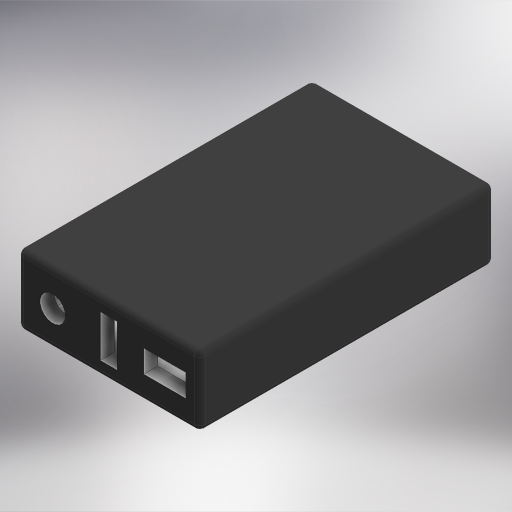
# Autodesk Inventor part: Lithium Battery
Saved by Autodesk Inventor 2024 (Build 280153000, 153)
## iProperties
Created: 2023-11-02
Part Number: Lithium Battery
Material: Genérico
Document SubType Name: Modeling
Designer: juesr
Density: 1 g/cm^3
Appearance: Valor por defecto
Author: juesr
Autodesk Inventor part; units mm, degrees
ref_plane "YZ Plane" through (0, 0, 0) normal (1, 0, 0) x (0, 1, 0)
ref_plane "XZ Plane" through (0, 0, 0) normal (0, 1, 0) x (-1, 0, 0)
ref_plane "XY Plane" through (0, 0, 0) normal (0, 0, 1) x (1, 0, 0)
sketch "Boceto1" plane through (0, 0, 0) normal (0, 1, 0) x (-1, 0, 0)
  line L0 (1.7308, 43.9183) -> (-63.2692, 43.9183)
  line L1 (-63.2692, 43.9183) -> (-63.2692, -61.0817)
  line L2 (-63.2692, -61.0817) -> (1.7308, -61.0817)
  line L3 (1.7308, -61.0817) -> (1.7308, 43.9183)
  point P0 (0, 0)
  dimension "d0" = 105
  dimension "d1" = 65
  constraints: 8 end point, 2 parallel, 1 horizontal, 1 perpendicular
  measures "d0" distance between parallel lines of L2 L0
  measures "d1" distance between parallel lines of L1 L3
extrude "Extrusión1" add sketch "Boceto1" along normal blind 25
shell "Vaciado1" thickness 5 removed faces 1 at (19.9359, 25, -26.0817)
sketch "Boceto2" plane through (0, 25, 0) normal (0, 1, 0) x (1, 0, 0)
  line L0 (3.2692, 56.0817) -> (3.2692, -38.9183) projected
  line L1 (58.2692, 56.0817) -> (3.2692, 56.0817)
  line L2 (3.2692, 56.0817) -> (3.2692, -38.9183)
  line L3 (3.2692, -38.9183) -> (58.2692, -38.9183)
  line L4 (58.2692, -38.9183) -> (58.2692, 56.0817)
  point P0 (0, 0)
  constraints: 8 end point, 2 parallel, 1 horizontal, 1 perpendicular
extrude "Extrusión2" add sketch "Boceto2" against normal blind 5
sketch "Boceto3" plane through (-1.7308, 0, 43.9183) normal (0, 0, 1) x (1, 0, 0)
  circle A0 centre (12.5, 12.5) radius 4.5
  line L0 (0, 0) -> (65, 0) projected
  line L1 (0, 0) -> (0, 25) projected
  point P0 (1.7308, 0)
  dimension "d12" = 9
  dimension "d13" = 12.5
  dimension "d14" = 12.5
  constraints: 1 centre point
  measures "d12" diameter of A0
  measures "d13" distance from line of L0 A0.centre
  measures "d14" distance from line of L1 A0.centre
extrude "Extrusión3" cut sketch "Boceto3" against normal blind 5
sketch "Boceto4" plane through (-1.7308, 0, 43.9183) normal (0, 0, 1) x (1, 0, 0)
  line L0 (60, 20) -> (5, 20) projected
  line L1 (60, 5) -> (5, 5) projected
  line L2 (29.5, 20) -> (35.5, 20)
  line L3 (35.5, 20) -> (35.5, 5)
  line L4 (35.5, 5) -> (29.5, 5)
  line L5 (29.5, 5) -> (29.5, 20)
  line L6 (0, 0) -> (0, 25) projected
  line L7 (65, 0) -> (65, 25) projected
  point P0 (1.7308, 0)
  point P1 (29.5, 12.5)
  point P2 (0, 12.5)
  dimension "d17" = 6
  dimension "d18" = 29.5
  dimension "d19" = 29.5
  constraints: 8 end point, 2 midpoint, 2 parallel, 2 point on line, 1 horizontal, 1 perpendicular
  measures "d17" distance from line of L3 point (29.5, 12.5)
  measures "d18" distance from line of point (0, 12.5) L5
  measures "d19" distance between parallel lines of L7 L3
extrude "Extrusión4" cut sketch "Boceto4" against normal blind 5
sketch "Boceto5" plane through (-1.7308, 0, 43.9183) normal (0, 0, 1) x (1, 0, 0)
  line L0 (45, 16.5) -> (60, 16.5)
  line L1 (60, 16.5) -> (60, 8.5)
  line L2 (60, 8.5) -> (45, 8.5)
  line L3 (45, 8.5) -> (45, 16.5)
  line L4 (0, 25) -> (65, 25) projected
  line L5 (0, 0) -> (65, 0) projected
  line L6 (65, 0) -> (65, 25) projected
  point P0 (1.7308, 0)
  point P1 (52.5, 8.5)
  point P2 (52.5, 16.5)
  point P3 (60, 12.5)
  point P4 (45, 12.5)
  point P5 (65, 12.5)
  dimension "d22" = 8
  dimension "d23" = 15
  dimension "d24" = 8.5
  dimension "d25" = 8.5
  dimension "d26" = 5
  constraints: 8 end point, 5 midpoint, 2 parallel, 1 horizontal, 1 perpendicular
  measures "d22" distance of point (52.5, 8.5) point (52.5, 16.5)
  measures "d23" distance of point (60, 12.5) point (45, 12.5)
  measures "d24" distance between parallel lines of L4 L0
  measures "d25" distance between parallel lines of L5 L2
  measures "d26" horizontal distance of point (65, 12.5) L0.end
extrude "Extrusión5" cut sketch "Boceto5" against normal blind 5
fillet "Empalme6" radius 2 1 edges at (-1.7308, 25, -8.5817)
fillet "Empalme7" radius 2 3 edges at (31.7692, 25, 43.9183) (-1.145, 24.4142, 43.9183) (-1.7308, 11.5, 43.9183)
fillet "Empalme8" radius 2 3 edges at (63.2692, 25, -9.5817) (63.2692, 24.4142, 43.3325) (63.2692, 11.5, 43.9183)
fillet "Empalme9" radius 2 5 edges at (30.7692, 25, -61.0817) (-1.145, 24.4142, -61.0817) (-1.7308, 11.5, -61.0817) (62.6834, 24.4142, -61.0817) (63.2692, 11.5, -61.0817)
fillet "Empalme10" radius 2 8 edges at (63.2692, 0, -8.5817) (62.6834, 0, -60.4959) (30.7692, 0, -61.0817) (-1.145, 0, -60.4959) (-1.7308, 0, -8.5817) (-1.145, 0, 43.3325) (30.7692, 0, 43.9183) (62.6834, 0, 43.3325)
